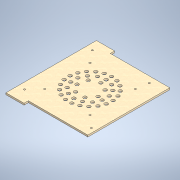
# Autodesk Inventor part: Platte2
Saved by Autodesk Inventor 2020 (Build 240168000, 168)
## iProperties
Created: 2022-03-24
Part Number: Platte2
Material: Pappel
Document SubType Name: Modeling
Designer: Eric
Density: 0.448 g/cm^3
Appearance: Pappel
Author: Eric
Autodesk Inventor part; units mm, degrees
ref_plane "YZ Plane" through (0, 0, 0) normal (1, 0, 0) x (0, 1, 0)
ref_plane "XZ Plane" through (0, 0, 0) normal (0, 1, 0) x (-1, 0, 0)
ref_plane "XY Plane" through (0, 0, 0) normal (0, 0, 1) x (1, 0, 0)
sketch "Skizze1" plane through (0, 0, 0) normal (0, 1, 0) x (-1, 0, 0)
  line L0 (0, 0) -> (180, 0)
  line L1 (180, 0) -> (180, -190)
  line L2 (180, -190) -> (0, -190)
  line L3 (0, -190) -> (0, 0)
  circle A0 centre (165.1, -18.17) radius 2 projected
  circle A1 centre (165.1, -175.65) radius 2 projected
  circle A2 centre (33.02, -175.65) radius 2 projected
  circle A3 centre (10.16, -18.17) radius 2 projected
  dimension "d0" = 190
  dimension "d1" = 180
  constraints: 8 end point, 2 parallel, 1 horizontal, 1 perpendicular
  measures "d0" distance between parallel lines of L2 L0
  measures "d1" distance of L1.end L2.end
extrude "Extrusion1" add sketch "Skizze1" along normal blind 4
sketch "Skizze2" plane through (0, 4, 0) normal (0, 1, 0) x (1, 0, 0)
  circle A0 centre (-90, 95) radius 95 construction
  line L0 (0, 190) -> (-180, 190) projected
  line L1 (-180, 0) -> (0, 0) projected
  circle A1 centre (-90, 95) radius 4 construction
  circle A2 centre (-90, 107.5) radius 4 construction
  circle A3 centre (-90, 120) radius 4
  circle A4 centre (-90, 132.5) radius 4
  circle A5 centre (-90, 145) radius 4
  line L2 (-180, 190) -> (-180, 0) projected
  line L3 (-180, 95) -> (0, 95) construction
  line L4 (0, 0) -> (0, 190) projected
  line L5 (-90, 145) -> (-90, 132.5) construction
  line L6 (-90, 132.5) -> (-90, 120) construction
  line L7 (-90, 120) -> (-90, 107.5) construction
  line L8 (-90, 107.5) -> (-90, 95) construction
  circle A6 centre (-104.7378, 142.7786) radius 4
  circle A7 centre (-118.166, 136.3119) radius 4
  circle A8 centre (-129.0916, 126.1745) radius 4
  circle A9 centre (-136.5437, 113.2671) radius 4
  circle A10 centre (-139.8602, 98.7365) radius 4
  circle A11 centre (-138.7464, 83.874) radius 4
  circle A12 centre (-133.3013, 70) radius 4
  circle A13 centre (-124.0086, 58.3474) radius 4
  circle A14 centre (-111.6942, 49.9516) radius 4
  circle A15 centre (-97.4521, 45.5585) radius 4
  circle A16 centre (-82.5479, 45.5585) radius 4
  circle A17 centre (-68.3058, 49.9516) radius 4
  circle A18 centre (-55.9914, 58.3474) radius 4
  circle A19 centre (-46.6987, 70) radius 4
  circle A20 centre (-41.2536, 83.874) radius 4
  circle A21 centre (-40.1398, 98.7365) radius 4
  circle A22 centre (-43.4563, 113.2671) radius 4
  circle A23 centre (-50.9084, 126.1745) radius 4
  circle A24 centre (-61.834, 136.3119) radius 4
  circle A25 centre (-106.2706, 128.7863) radius 4
  circle A26 centre (-119.3187, 118.3809) radius 4
  circle A27 centre (-126.5598, 103.3445) radius 4
  circle A28 centre (-126.5598, 86.6555) radius 4
  circle A29 centre (-119.3187, 71.6191) radius 4
  circle A30 centre (-106.2706, 61.2137) radius 4
  circle A31 centre (-90, 57.5) radius 4
  circle A32 centre (-73.7294, 61.2137) radius 4
  circle A33 centre (-60.6813, 71.6191) radius 4
  circle A34 centre (-53.4402, 86.6555) radius 4
  circle A35 centre (-53.4402, 103.3445) radius 4
  circle A36 centre (-60.6813, 118.3809) radius 4
  circle A37 centre (-73.7294, 128.7863) radius 4
  circle A38 centre (-109.5458, 110.5872) radius 4
  circle A39 centre (-114.3732, 89.437) radius 4
  circle A40 centre (-100.8471, 72.4758) radius 4
  circle A41 centre (-79.1529, 72.4758) radius 4
  circle A42 centre (-65.6268, 89.437) radius 4
  circle A43 centre (-70.4542, 110.5872) radius 4
  circle A44 centre (-75.2622, 142.7786) radius 4
  circle A45 centre (-37.5, 147.5) radius 2
  circle A46 centre (-37.5, 42.5) radius 2
  circle A47 centre (-142.5, 42.5) radius 2
  circle A48 centre (-142.5, 147.5) radius 2
  line L9 (-142.5, 147.5) -> (-37.5, 147.5) construction
  line L10 (-37.5, 147.5) -> (-37.5, 42.5) construction
  line L11 (-37.5, 42.5) -> (-142.5, 42.5) construction
  line L12 (-142.5, 42.5) -> (-142.5, 147.5) construction
  line L13 (-90, 147.5) -> (-90, 95) construction
  line L14 (-90, 95) -> (-37.5, 95) construction
  dimension "d4" = 8
  dimension "d5" = 50
  dimension "d8" = 360
  dimension "d12" = 360
  dimension "d16" = 360
  dimension "d20" = 4
  dimension "d21" = 105
  constraints: 49 centre point, 22 end point, 8 equal length, 7 equal radius, 5 midpoint, 4 perpendicular, 2 tangent, 2 vertical, 1 coincident, 87 other
  measures "d4" diameter of A1
  measures "d5" distance from line of L3 L5.start
  measures "d20" diameter of A45
  measures "d21" distance of L9.end L10.end
extrude "Extrusion2" cut sketch "Skizze2" against normal blind 4 contours A3 | A4 | A5 | A6 | A7 | A8 | A9 | A10 | A11 | A12 | A13 | A14 | A15 | A16 | A17 | A18 | A19 | A20 | A21 | A22 | A23 | A24 | A25 | A26 | A27 | A28 | A29 | A30 | A31 | A32 | A33 | A34 | A35 | A36 | A37 | A38 | A39 | A40 | A41 | A42 | A43 | A44 | A45 | A46 | A47 | A48
sketch "Skizze3" plane through (0, 0, 0) normal (0, -1, 0) x (1, 0, 0)
  line L0 (0, -190) -> (-180, -190) projected
  line L1 (-180, -190) -> (-138, -190)
  line L2 (-138, -190) -> (-138, -200)
  line L3 (-138, -200) -> (-180, -200)
  line L4 (-180, -200) -> (-180, -190)
  line L5 (-180, 0) -> (-138, 0)
  line L6 (-138, 0) -> (-138, 10)
  line L7 (-138, 10) -> (-180, 10)
  line L8 (-180, 10) -> (-180, 0)
  line L9 (0, 0) -> (0, -190) projected
  dimension "d22" = 10
  dimension "d23" = 138
  constraints: 16 end point, 4 parallel, 2 equal length, 2 horizontal, 2 perpendicular
  measures "d22" distance of L3.end L0.end
  measures "d23" distance between parallel lines of L9 L6
extrude "Extrusion3" add sketch "Skizze3" against normal blind 4
